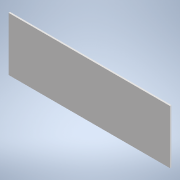
# Autodesk Inventor part: PrimaryCoilFerriteLayer
Saved by Autodesk Inventor 2021 (Build 250183000, 183)
## iProperties
Created: 2022-01-19
Part Number: PrimaryCoilFerriteLayer
Material: Iron, Cast
Document SubType Name: Modeling
Designer: avan411
Density: 7.15 g/cm^3
Appearance: Iron Gray
Author: avan411
Autodesk Inventor part; units mm, degrees
ref_plane "YZ Plane" through (0, 0, 0) normal (1, 0, 0) x (0, 1, 0)
ref_plane "XZ Plane" through (0, 0, 0) normal (0, 1, 0) x (-1, 0, 0)
ref_plane "XY Plane" through (0, 0, 0) normal (0, 0, 1) x (1, 0, 0)
sketch "Sketch1" plane through (0, 0, 0) normal (0, 0, 1) x (1, 0, 0)
  line L0 (97.5839, -20.2585) -> (97.5839, -84.5585) construction
  line L1 (97.5839, -52.4085) -> (19.6066, -52.4085)
  line L2 (622.5839, -227.4085) -> (-427.4161, -227.4085)
  line L3 (-427.4161, -227.4085) -> (-427.4161, 122.5915)
  line L4 (-427.4161, 122.5915) -> (622.5839, 122.5915)
  line L5 (622.5839, 122.5915) -> (622.5839, -227.4085)
  line L6 (622.5839, -227.4085) -> (-427.4161, 122.5915) construction
  line L7 (-427.4161, -227.4085) -> (622.5839, 122.5915) construction
  line L8 (122.536, -54.5185) -> (122.536, 53.9215) projected
  line L9 (122.536, 53.9215) -> (107.7839, 53.9215) projected
  line L10 (107.7839, 53.9215) -> (107.7839, -54.5185) projected
  line L11 (107.7839, -54.5185) -> (122.536, -54.5185) projected
  line L12 (122.5839, -162.9585) -> (122.5839, -54.5185) projected
  line L13 (122.5839, -54.5185) -> (107.7839, -54.5185) projected
  line L14 (107.7839, -54.5185) -> (107.7839, -162.9585) projected
  line L15 (107.7839, -162.9585) -> (122.5839, -162.9585) projected
  line L16 (12.536, -54.5185) -> (12.536, 53.9215) projected
  line L17 (12.536, 53.9215) -> (-2.2161, 53.9215) projected
  line L18 (-2.2161, 53.9215) -> (-2.2161, -54.5185) projected
  line L19 (-2.2161, -54.5185) -> (12.536, -54.5185) projected
  line L20 (12.5839, -162.9585) -> (12.5839, -54.5185) projected
  line L21 (12.5839, -54.5185) -> (-2.2161, -54.5185) projected
  line L22 (-2.2161, -54.5185) -> (-2.2161, -162.9585) projected
  line L23 (-2.2161, -162.9585) -> (12.5839, -162.9585) projected
  line L24 (-97.4161, -162.9585) -> (-97.4161, -54.5185) projected
  line L25 (-97.4161, -54.5185) -> (-112.2161, -54.5185) projected
  line L26 (-112.2161, -54.5185) -> (-112.2161, -162.9585) projected
  line L27 (-112.2161, -162.9585) -> (-97.4161, -162.9585) projected
  line L28 (-97.464, -54.5185) -> (-97.464, 53.9215) projected
  line L29 (-97.464, 53.9215) -> (-112.2161, 53.9215) projected
  line L30 (-112.2161, 53.9215) -> (-112.2161, -54.5185) projected
  line L31 (-112.2161, -54.5185) -> (-97.464, -54.5185) projected
  line L32 (-317.464, -54.5185) -> (-317.464, 53.9215) projected
  line L33 (-317.464, 53.9215) -> (-332.2161, 53.9215) projected
  line L34 (-332.2161, 53.9215) -> (-332.2161, -54.5185) projected
  line L35 (-332.2161, -54.5185) -> (-317.464, -54.5185) projected
  line L36 (-317.4161, -162.9585) -> (-317.4161, -54.5185) projected
  line L37 (-317.4161, -54.5185) -> (-332.2161, -54.5185) projected
  line L38 (-332.2161, -54.5185) -> (-332.2161, -162.9585) projected
  line L39 (-332.2161, -162.9585) -> (-317.4161, -162.9585) projected
  line L40 (-207.4161, -162.9585) -> (-207.4161, -54.5185) projected
  line L41 (-207.4161, -54.5185) -> (-222.2161, -54.5185) projected
  line L42 (-222.2161, -54.5185) -> (-222.2161, -162.9585) projected
  line L43 (-222.2161, -162.9585) -> (-207.4161, -162.9585) projected
  line L44 (-207.464, -54.5185) -> (-207.464, 53.9215) projected
  line L45 (-207.464, 53.9215) -> (-222.2161, 53.9215) projected
  line L46 (-222.2161, 53.9215) -> (-222.2161, -54.5185) projected
  line L47 (-222.2161, -54.5185) -> (-207.464, -54.5185) projected
  line L48 (562.536, -54.5185) -> (562.536, 53.9215) projected
  line L49 (562.536, 53.9215) -> (547.7839, 53.9215) projected
  line L50 (547.7839, 53.9215) -> (547.7839, -54.5185) projected
  line L51 (547.7839, -54.5185) -> (562.536, -54.5185) projected
  line L52 (562.5839, -162.9585) -> (562.5839, -54.5185) projected
  line L53 (562.5839, -54.5185) -> (547.7839, -54.5185) projected
  line L54 (547.7839, -54.5185) -> (547.7839, -162.9585) projected
  line L55 (547.7839, -162.9585) -> (562.5839, -162.9585) projected
  line L56 (452.5839, -162.9585) -> (452.5839, -54.5185) projected
  line L57 (452.5839, -54.5185) -> (437.7839, -54.5185) projected
  line L58 (437.7839, -54.5185) -> (437.7839, -162.9585) projected
  line L59 (437.7839, -162.9585) -> (452.5839, -162.9585) projected
  line L60 (452.536, -54.5185) -> (452.536, 53.9215) projected
  line L61 (452.536, 53.9215) -> (437.7839, 53.9215) projected
  line L62 (437.7839, 53.9215) -> (437.7839, -54.5185) projected
  line L63 (437.7839, -54.5185) -> (452.536, -54.5185) projected
  line L64 (342.536, -54.5185) -> (342.536, 53.9215) projected
  line L65 (342.536, 53.9215) -> (327.7839, 53.9215) projected
  line L66 (327.7839, 53.9215) -> (327.7839, -54.5185) projected
  line L67 (327.7839, -54.5185) -> (342.536, -54.5185) projected
  line L68 (342.5839, -162.9585) -> (342.5839, -54.5185) projected
  line L69 (342.5839, -54.5185) -> (327.7839, -54.5185) projected
  line L70 (327.7839, -54.5185) -> (327.7839, -162.9585) projected
  line L71 (327.7839, -162.9585) -> (342.5839, -162.9585) projected
  line L72 (232.536, -54.5185) -> (232.536, 53.9215) projected
  line L73 (232.536, 53.9215) -> (217.7839, 53.9215) projected
  line L74 (217.7839, 53.9215) -> (217.7839, -54.5185) projected
  line L75 (217.7839, -54.5185) -> (232.536, -54.5185) projected
  line L76 (232.5839, -162.9585) -> (232.5839, -54.5185) projected
  line L77 (232.5839, -54.5185) -> (217.7839, -54.5185) projected
  line L78 (217.7839, -54.5185) -> (217.7839, -162.9585) projected
  line L79 (217.7839, -162.9585) -> (232.5839, -162.9585) projected
  line L80 (144.8839, -131.8585) -> (144.8839, -227.4085) projected
  line L81 (140.5839, -227.4085) -> (140.5839, -131.8585) projected
  arc A0 (144.8839, -131.8585) -> (97.5839, -84.5585) centre (97.5839, -131.8585) ccw projected
  arc A1 (140.5839, -131.8585) -> (97.5839, -88.8585) centre (97.5839, -131.8585) ccw projected
  line L82 (-34.764, -227.4085) -> (-34.764, -63.2585) projected
  line L83 (-30.464, -63.2585) -> (-30.464, -227.4085) projected
  arc A2 (12.536, -20.2585) -> (-30.464, -63.2585) centre (12.536, -63.2585) ccw projected
  arc A3 (12.536, -15.9585) -> (-34.764, -63.2585) centre (12.536, -63.2585) ccw projected
  circle A4 centre (-417.4161, 112.5915) radius 3 projected
  line L84 (622.5839, 122.5915) -> (-427.4161, 122.5915) projected
  line L85 (622.5839, -227.4085) -> (622.5839, 122.5915) projected
  line L86 (-427.4161, -227.4085) -> (622.5839, -227.4085) projected
  line L87 (-427.4161, 122.5915) -> (-427.4161, -227.4085) projected
  circle A5 centre (-417.4161, -217.4085) radius 3 projected
  line L88 (622.5839, 122.5915) -> (-427.4161, 122.5915) projected
  line L89 (622.5839, -227.4085) -> (622.5839, 122.5915) projected
  line L90 (-427.4161, -227.4085) -> (622.5839, -227.4085) projected
  line L91 (-427.4161, 122.5915) -> (-427.4161, -227.4085) projected
  line L92 (622.5839, 122.5915) -> (-427.4161, 122.5915) projected
  line L93 (622.5839, -227.4085) -> (622.5839, 122.5915) projected
  line L94 (-427.4161, -227.4085) -> (622.5839, -227.4085) projected
  line L95 (-427.4161, 122.5915) -> (-427.4161, -227.4085) projected
  circle A6 centre (612.5839, 112.5915) radius 3 projected
  circle A7 centre (612.5839, -217.4085) radius 3 projected
  circle A8 centre (-159.9161, -217.4085) radius 3 projected
  circle A9 centre (97.5839, -217.4085) radius 3 projected
  circle A10 centre (355.0839, -217.4085) radius 3 projected
  circle A11 centre (-159.9161, 112.5915) radius 3 projected
  circle A12 centre (97.5839, 112.5915) radius 3 projected
  circle A13 centre (355.0839, 112.5915) radius 3 projected
  circle A14 centre (97.5839, 112.5915) radius 3 projected
  circle A15 centre (612.5839, -217.4085) radius 3 projected
  circle A16 centre (355.0839, -217.4085) radius 3 projected
  circle A17 centre (97.5839, -217.4085) radius 3 projected
  circle A18 centre (-159.9161, -217.4085) radius 3 projected
  circle A19 centre (-417.4161, -217.4085) radius 3 projected
  circle A20 centre (355.0839, 112.5915) radius 3 projected
  circle A21 centre (-417.4161, 112.5915) radius 3 projected
  circle A22 centre (612.5839, 112.5915) radius 3 projected
  circle A23 centre (-159.9161, 112.5915) radius 3 projected
  circle A24 centre (97.5839, 112.5915) radius 3 projected
  circle A25 centre (612.5839, -217.4085) radius 3 projected
  circle A26 centre (355.0839, -217.4085) radius 3 projected
  circle A27 centre (97.5839, -217.4085) radius 3 projected
  circle A28 centre (-159.9161, -217.4085) radius 3 projected
  circle A29 centre (-417.4161, -217.4085) radius 3 projected
  circle A30 centre (355.0839, 112.5915) radius 3 projected
  circle A31 centre (-417.4161, 112.5915) radius 3 projected
  circle A32 centre (612.5839, 112.5915) radius 3 projected
  circle A33 centre (-159.9161, 112.5915) radius 3 projected
  circle A34 centre (97.5839, 112.5915) radius 3 projected
  circle A35 centre (612.5839, -217.4085) radius 3 projected
  circle A36 centre (355.0839, -217.4085) radius 3 projected
  circle A37 centre (97.5839, -217.4085) radius 3 projected
  circle A38 centre (-159.9161, -217.4085) radius 3 projected
  circle A39 centre (-417.4161, -217.4085) radius 3 projected
  circle A40 centre (355.0839, 112.5915) radius 3 projected
  circle A41 centre (-417.4161, 112.5915) radius 3 projected
  circle A42 centre (612.5839, 112.5915) radius 3 projected
  circle A43 centre (-159.9161, 112.5915) radius 3 projected
  point P0 (0, 0)
  point P1 (-2.2161, -18.3178)
  point P2 (-2.2161, -22.8682)
  point P3 (122.5839, -96.8728)
  point P4 (122.5839, -91.7052)
  dimension "d0" = 1050
  dimension "d1" = 350
  constraints: 16 end point, 3 midpoint, 2 parallel, 1 horizontal, 1 perpendicular
  measures "d0" distance of L3.end L4.end
  measures "d1" distance of L2.end L3.end
extrude "Extrusion2" add sketch "Sketch1" along normal blind 8.5 contours L2 L80 A0 L12 L13 L8 L9 L10 L14 L15 A1 L81 L83 A2 L18 L22 L23 L20 L21 L16 L17 A3 L82 L3 L4 L5
body "Solid2"
